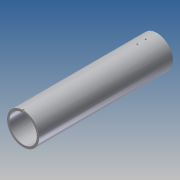
# Autodesk Inventor part: 2h2slv
Saved by Autodesk Inventor 2014 SP1 (Build 180222100, 222)
## iProperties
Company: HERA Project
Created: 2013-05-14
Part Number: 2h2slv
Material: PVC-Piping
Document SubType Name: Modeling
Designer: David DeBoer
Density: 1.4 g/cm^3
Mass: 429.807 g
Surface Area: 1214.86 cm^2
Volume: 307.005 cm^3
Description: Hub mating sleeve
Appearance: Smooth - White
Author: David DeBoer
Title: Hub mating sleeve
Autodesk Inventor part; units mm, degrees
ref_plane "YZ Plane" through (0, 0, 0) normal (1, 0, 0) x (0, 1, 0)
ref_plane "XZ Plane" through (0, 0, 0) normal (0, 1, 0) x (-1, 0, 0)
ref_plane "XY Plane" through (0, 0, 0) normal (0, 0, 1) x (1, 0, 0)
sketch "Sketch1" plane through (0, 0, 0) normal (0, 0, 1) x (1, 0, 0)
  circle A0 centre (0, 0) radius 36.5125
  circle A1 centre (0, 0) radius 31.3563
  dimension "d0" = 73.025
  dimension "d2" = 5.1562
  constraints: 2 centre point, 1 coincident
  measures "d0" diameter of A0
  measures "d2" radial gap between concentric circles of A1 A0
extrude "Extrusion1" add sketch "Sketch1" along normal blind 304.8
sketch "Sketch2" plane through (0, 0, 304.8) normal (0, 0, 1) x (1, 0, 0)
  circle A0 centre (0, 0) radius 31.3563 projected
  circle A1 centre (0, 0) radius 36.5125 projected
  point P0 (0, 36.5125)
  constraints: 1 vertical alignment, 1 other
ref_plane "Work Plane1" through (0, 36.5125, 304.8) normal (0, 1, 0) x (-1, 0, 0)
sketch "Sketch5" plane through (0, 36.5125, 304.8) normal (0, 1, 0) x (-1, 0, 0)
  circle A0 centre (0, -279.4) radius 4.4901
  circle A1 centre (0, -260.35) radius 4.4901
  point P0 (0, -304.8)
  dimension "d25" = 25.4
  dimension "d26" = 19.05
  constraints: 2 centre point
  measures "d25" distance of point (0, -304.8) A0.centre
  measures "d26" distance of A0.centre A1.centre
hole "Hole3" at (0, 36.5125, 44.45) at (0, 36.5125, 25.4) direction (0, -1, 0) diameter 3.175 end through all
sketch "Sketch6" plane through (0, 0, 304.8) normal (0, 0, 1) x (1, 0, 0)
  circle A0 centre (0, 0) radius 31.3563 projected
  circle A1 centre (0, 0) radius 36.5125 projected
  point P0 (0, 36.5125)
  constraints: 1 vertical alignment, 1 other
ref_plane "Work Plane2" through (0, 36.5125, 304.8) normal (0, 1, 0) x (-1, 0, 0)
sketch "Sketch8" plane through (0, 36.5125, 304.8) normal (0, 1, 0) x (-1, 0, 0)
  line L0 (-1.27, 0) -> (1.27, 0)
  line L1 (1.27, 0) -> (1.27, -2.54)
  line L2 (1.27, -2.54) -> (-1.27, -2.54)
  line L3 (-1.27, -2.54) -> (-1.27, 0)
  line L4 (0, 0) -> (0, -2.54) construction
  point P0 (0, -304.8)
  dimension "d34" = 2.54
  dimension "d35" = 2.54
  constraints: 10 end point, 2 midpoint, 2 parallel, 1 coincident, 1 horizontal, 1 perpendicular
  measures "d34" distance of L1.end L2.end
  measures "d35" distance of L0.end L1.end
extrude "Extrusion2" cut sketch "Sketch8" against normal blind 2.54
body "Solid1"
